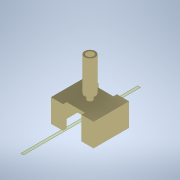
# Autodesk Inventor part: end_effector_clamp
Saved by Autodesk Inventor 2020 (Build 240168000, 168)
## iProperties
Created: 2020-07-03
Part Number: end_effector_clamp
Material: Generic
Document SubType Name: Modeling
Designer: Ashiqrahman
Density: 1 g/cm^3
Appearance: Gold - Metal
Author: Ashiqrahman
Autodesk Inventor part; units mm, degrees
ref_plane "YZ Plane" through (0, 0, 0) normal (1, 0, 0) x (0, 1, 0)
ref_plane "XZ Plane" through (0, 0, 0) normal (0, 1, 0) x (-1, 0, 0)
ref_plane "XY Plane" through (0, 0, 0) normal (0, 0, 1) x (1, 0, 0)
ref_plane "Work Plane1" through (53.4484, -39.2696, -18.6043) normal (0, -1, 0) x (1, 0, 0)
sketch "Sketch1" plane through (53.4484, -39.2696, -18.6043) normal (0, -1, 0) x (1, 0, 0)
  line L0 (-60, -100) -> (60, -100)
  line L1 (60, -100) -> (60, 50)
  line L2 (60, 50) -> (-60, 50)
  line L3 (-60, 50) -> (-60, -100)
  line L4 (-60, -100) -> (60, 50) construction
  line L5 (60, -100) -> (-60, 50) construction
  line L6 (60, 50) -> (50, 50)
  line L7 (50, 50) -> (50, -100)
  line L8 (50, -100) -> (60, -100)
  line L9 (60, -100) -> (60, 50)
  line L10 (-60, -100) -> (-50, -100)
  line L11 (-50, -100) -> (-50, 50)
  line L12 (-50, 50) -> (-60, 50)
  line L13 (-60, 50) -> (-60, -100)
  line L14 (-30, 150) -> (-30, -150) projected
  line L15 (21.7735, 150) -> (21.7735, -150) projected
  line L16 (60, 50) -> (21.7735, 50)
  line L17 (21.7735, 50) -> (21.7735, 40)
  line L18 (21.7735, 40) -> (60, 40)
  line L19 (60, 40) -> (60, 50)
  line L20 (60, -100) -> (21.7735, -100)
  line L21 (21.7735, -100) -> (21.7735, -90)
  line L22 (21.7735, -90) -> (60, -90)
  line L23 (60, -90) -> (60, -100)
  line L24 (-60, 50) -> (-30, 50)
  line L25 (-30, 50) -> (-30, 40)
  line L26 (-30, 40) -> (-60, 40)
  line L27 (-60, 40) -> (-60, 50)
  line L28 (-60, -100) -> (-30, -100)
  line L29 (-30, -100) -> (-30, -90)
  line L30 (-60, -40) -> (-60, -100)
  line L31 (-30, 150) -> (-30, -150) projected
  line L32 (-60, -40) -> (-30, -40)
  line L33 (-30, -100) -> (-30, -40)
  line L34 (-30, 50) -> (-30, 40)
  point P0 (-53.4484, 18.6043)
  point P1 (0, -25)
  point P2 (-50, 40)
  point P3 (-30, 50)
  point P4 (50, 40)
  point P5 (50, -90)
  point P6 (21.7735, -100)
  point P7 (21.7735, 50)
  point P8 (0, -25)
  dimension "d0" = 120
  dimension "d1" = 150
  dimension "d2" = 10
  dimension "d3" = 10
  dimension "d4" = 10
  dimension "d5" = 10
  dimension "d6" = 10
  dimension "d7" = 10
  dimension "d13" = 75
  dimension "d14" = 0
  constraints: 64 end point, 13 parallel, 13 point on line, 8 perpendicular, 7 horizontal, 2 midpoint, 1 collinear
  measures "d0" distance of L2.end L1.end
  measures "d1" distance of L1.end L0.end
  measures "d2" distance of L8.end L7.end
  measures "d3" distance of L12.end L11.end
  measures "d4" distance of L17.end L16.end
  measures "d5" distance of L20.end L21.end
  measures "d6" distance of L24.end L25.end
  measures "d7" distance of L29.end L28.end
  measures "d13" distance from line of L2 point (0, -25)
  measures "d14" distance of point (0, -25) point (0, -25)
extrude "Extrusion1" add sketch "Sketch1" against normal blind 65 contours L3 L32 L11 L0 | L11 L32 L14 L0 | L3 L26 L11 L32 | L11 L26 L14 L32 | L3 L2 L11 L26 | L15 L22 L7 L0 | L11 L2 L14 L26 | L7 L22 L1 L0 | L7 L18 L1 L22 | L15 L2 L7 L18 | L7 L2 L1 L18
sketch "Sketch2" plane through (103.4484, -39.2696, -108.6043) normal (-1, 0, 0) x (0, 0, 1)
  line L0 (0, 65) -> (130, 65) projected
  line L1 (130, 0) -> (130, 65) projected
  line L2 (0, 65) -> (130, 65)
  line L3 (130, 65) -> (130, 55)
  line L4 (130, 55) -> (0, 55)
  line L5 (0, 55) -> (0, 65)
  point P0 (108.6043, 39.2696)
  dimension "d10" = 10
  constraints: 8 end point, 2 parallel, 1 horizontal, 1 perpendicular, 1 point on line
  measures "d10" distance of L2.end L3.end
extrude "Extrusion2" [suppressed]
sketch "Sketch3" plane through (53.4484, 25.7304, -18.6043) normal (0, 1, 0) x (1, 0, 0)
  point P0 (-53.4484, -18.6043)
sketch "Sketch4" plane through (53.4484, 25.7304, -18.6043) normal (0, 1, 0) x (1, 0, 0)
  point P0 (-53.4484, -18.6043)
body "Solid1"
